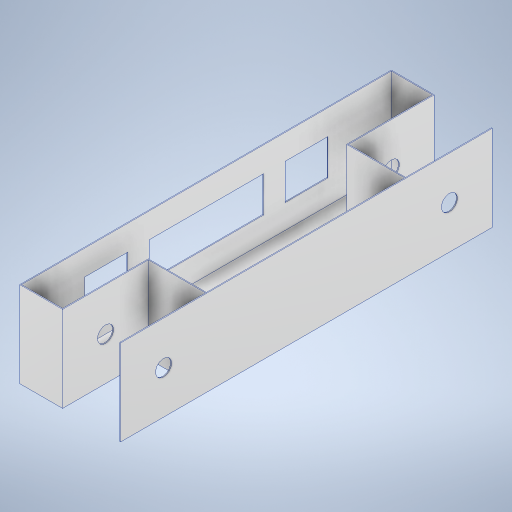
# Autodesk Inventor part: DriveHousing
Saved by Autodesk Inventor 2023 (Build 270158000, 158)
## iProperties
Created: 2022-09-20
Part Number: DriveHousing
Material: Aluminum 6061
Document SubType Name: Modeling
Designer: seene
Density: 2.7 g/cm^3
Appearance: Aluminum - Flat
Author: seene
Autodesk Inventor part; units mm, degrees
ref_plane "YZ Plane" through (0, 0, 0) normal (1, 0, 0) x (0, 1, 0)
ref_plane "XZ Plane" through (0, 0, 0) normal (0, 1, 0) x (-1, 0, 0)
ref_plane "XY Plane" through (0, 0, 0) normal (0, 0, 1) x (1, 0, 0)
sketch "Sketch1" plane through (0, 0, 0) normal (0, 1, 0) x (-1, 0, 0)
  line L0 (0, 0) -> (-76.2, 0)
  line L1 (-76.2, 0) -> (-76.2, -152.4)
  line L2 (-76.2, -152.4) -> (-177.8, -152.4)
  line L3 (0, -660.4) -> (-76.2, -660.4)
  line L4 (-76.2, -660.4) -> (-76.2, -508)
  line L5 (-76.2, -508) -> (-177.8, -508)
  line L6 (0, 0) -> (0, -660.4)
  line L7 (-177.8, -152.4) -> (-177.8, -508)
  dimension "d4" = 660.4
  dimension "d91" = 152.4
  dimension "d92" = 152.4
  dimension "d95" = 177.8
  dimension "d96" = 101.6
  dimension "d97" = 101.6
  dimension "d98" = 177.8
  constraints: 18 end point, 4 horizontal, 2 vertical, 1 perpendicular
  measures "d4" distance of L0.start L3.start
  measures "d91" distance of L0.end L1.end
  measures "d92" distance of L3.end L4.end
  measures "d95" distance from line of L2.end L6
  measures "d96" distance of L4.end L5.end
  measures "d97" distance of L1.end L2.end
  measures "d98" horizontal distance of L5.end L3.start
extrude "Extrusion1" add sketch "Sketch1" along normal blind 1.5875
sketch "Sketch3" plane through (0, 1.5875, 0) normal (0, 1, 0) x (1, 0, 0)
  line L0 (0, 0) -> (76.2, 0) projected
  line L1 (76.2, 0) -> (76.2, 152.4) projected
  line L2 (76.2, 152.4) -> (177.8, 152.4) projected
  line L3 (177.8, 152.4) -> (177.8, 508) projected
  line L4 (177.8, 508) -> (76.2, 508) projected
  line L5 (76.2, 508) -> (76.2, 660.4) projected
  line L6 (76.2, 660.4) -> (0, 660.4) projected
  line L7 (0, 660.4) -> (0, 0) projected
  line L8 (1.5875, 658.8125) -> (74.6125, 658.8125)
  line L9 (74.6125, 658.8125) -> (74.6125, 506.4125)
  line L10 (74.6125, 506.4125) -> (177.8, 506.4125)
  line L11 (177.8, 153.9875) -> (74.6125, 153.9875)
  line L12 (74.6125, 153.9875) -> (74.6125, 1.5875)
  line L13 (74.6125, 1.5875) -> (1.5875, 1.5875)
  line L14 (1.5875, 1.5875) -> (1.5875, 658.8125)
  line L15 (177.8, 0) -> (179.3875, 0)
  line L16 (179.3875, 0) -> (179.3875, 660.4)
  line L17 (179.3875, 660.4) -> (177.8, 660.4)
  line L18 (177.8, 660.4) -> (177.8, 0)
  dimension "d114" = 1.5875
  dimension "d115" = 1.5875
  dimension "d116" = 1.5875
  constraints: 22 end point, 2 parallel, 2 point on line, 1 collinear, 1 horizontal, 1 perpendicular, 5 other
  measures "d114" distance between parallel lines of L6 L8
  measures "d115" distance of L17.end L16.end
  measures "d116" distance between parallel lines of L11 L2
extrude "Extrusion4" add sketch "Sketch3" along normal blind 150.8125 contours L7 L6 L5 L4 L3 L10 L9 L8 L14 L13 L12 L11 L2 L1 L0
sketch "Sketch6" plane through (0, 0, -660.4) normal (-1, 0, 0) x (0, 0, 1)
  line L0 (330.2, 152.4) -> (330.2, 0) construction
  line L1 (0, 76.2) -> (660.4, 76.2) construction
  line L2 (228.6, 44.45) -> (431.8, 44.45)
  line L3 (431.8, 44.45) -> (431.8, 107.95)
  line L4 (431.8, 107.95) -> (228.6, 107.95)
  line L5 (228.6, 107.95) -> (228.6, 44.45)
  line L6 (228.6, 44.45) -> (431.8, 107.95) construction
  line L7 (431.8, 44.45) -> (228.6, 107.95) construction
  line L8 (190.5, 44.45) -> (114.3, 44.45)
  line L9 (114.3, 44.45) -> (114.3, 107.95)
  line L10 (114.3, 107.95) -> (190.5, 107.95)
  line L11 (190.5, 107.95) -> (190.5, 44.45)
  line L12 (190.5, 44.45) -> (114.3, 107.95) construction
  line L13 (114.3, 44.45) -> (190.5, 107.95) construction
  line L14 (469.9, 44.45) -> (546.1, 44.45)
  line L15 (546.1, 44.45) -> (546.1, 107.95)
  line L16 (546.1, 107.95) -> (469.9, 107.95)
  line L17 (469.9, 107.95) -> (469.9, 44.45)
  line L18 (469.9, 44.45) -> (546.1, 107.95) construction
  line L19 (546.1, 44.45) -> (469.9, 107.95) construction
  line L20 (0, 152.4) -> (660.4, 152.4) projected
  line L21 (0, 0) -> (0, 152.4) projected
  point P0 (330.2, 76.2)
  point P1 (152.4, 76.2)
  point P2 (508, 76.2)
  dimension "d21" = 203.2
  dimension "d22" = 63.5
  dimension "d23" = 76.2
  dimension "d24" = 63.5
  dimension "d25" = 38.1
  dimension "d26" = 76.2
  dimension "d27" = 63.5
  dimension "d28" = 38.1
  constraints: 40 end point, 10 midpoint, 6 parallel, 4 horizontal, 4 perpendicular, 2 point on line, 1 vertical
  measures "d21" distance of L4.end L3.end
  measures "d22" distance of L3.end L2.end
  measures "d23" distance of L9.end L10.end
  measures "d24" distance of L8.end L9.end
  measures "d25" distance between parallel lines of L5 L11
  measures "d26" distance of L16.end L15.end
  measures "d27" distance of L15.end L14.end
  measures "d28" distance between parallel lines of L3 L17
extrude "Extrusion6" add sketch "Sketch3" along normal blind 150.8125 and the other way blind 1.5875 contours L3 L18 L17 L16 L15
extrude "Extrusion7" cut sketch "Sketch6" against normal up to surface (1.5875 mm away)
sketch "Sketch8" plane through (179.3875, 0, -660.4) normal (1, 0, 0) x (0, 0, -1)
  circle A0 centre (-584.2, 76.2) radius 14.2875
  circle A1 centre (-76.2, 76.2) radius 14.2875
  line L0 (-660.4, 152.4) -> (0, 152.4) projected
  line L1 (-660.4, 0) -> (-660.4, 152.4) projected
  line L2 (0, 0) -> (0, 152.4) projected
  dimension "d117" = 28.575
  dimension "d118" = 28.575
  dimension "d119" = 76.2
  dimension "d120" = 76.2
  dimension "d121" = 76.2
  dimension "d122" = 76.2
  constraints: 2 centre point
  measures "d117" diameter of A0
  measures "d118" diameter of A1
  measures "d119" distance from line of L0 A0.centre
  measures "d120" distance from line of L1 A0.centre
  measures "d121" distance from line of L2 A1.centre
  measures "d122" distance from line of A1.centre L0
extrude "Extrusion9" cut sketch "Sketch8" against normal up to surface (104.775 mm away)
equation "\"d96\" = d97"
equation "\"d98\" = d95"
equation "\"d24\" = d22"
equation "\"d27\" = d22"
equation "\"d28\" = d25"
body "Solid1"
